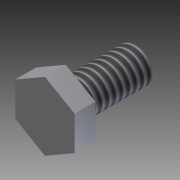
# Autodesk Inventor part: Bolt .5 1764
Saved by Autodesk Inventor 2011 (Build 150239000, 239)
## iProperties
Created: 2010-01-27
Part Number: Bolt .5 1764
Document SubType Name: Modeling
Designer: jgehrig
Density: 1 g/cm^3
Author: jgehrig
Autodesk Inventor part; units mm, degrees
ref_plane "YZ Plane" through (0, 0, 0) normal (1, 0, 0) x (0, 1, 0)
ref_plane "XZ Plane" through (0, 0, 0) normal (0, 1, 0) x (-1, 0, 0)
ref_plane "XY Plane" through (0, 0, 0) normal (0, 0, 1) x (1, 0, 0)
sketch "Sketch1" plane through (0, 0, 0) normal (0, 0, 1) x (1, 0, 0)
  circle A0 centre (0, 0) radius 3.175
  dimension "d0" = 6.35
  constraints: 1 centre point, 1 coincident
  measures "d0" diameter of A0
extrude "Extrusion1" add sketch "Sketch1" along normal blind 12.7
sketch "Sketch2" plane through (0, 0, 12.7) normal (0, 0, 1) x (1, 0, 0)
  circle A0 centre (0, 0) radius 3.175 projected
  line L0 (0, 6.2325) -> (5.3975, 3.1162)
  line L1 (5.3975, 3.1162) -> (5.3975, -3.1162)
  line L2 (5.3975, -3.1162) -> (0, -6.2325)
  line L3 (0, -6.2325) -> (-5.3975, -3.1162)
  line L4 (-5.3975, -3.1162) -> (-5.3975, 3.1162)
  line L5 (-5.3975, 3.1162) -> (0, 6.2325)
  dimension "d3" = 10.795
  constraints: 12 end point, 1 coincident, 13 other
  measures "d3" distance between parallel lines of L1 L4
extrude "Extrusion2" add sketch "Sketch2" along normal blind 3.81 contours A0 | L0 L1 L2 L3 L4 L5
thread "Thread1" size "1/4-20 UNC" class "2A" standard "ANSI Unified Screw Threads" full length
body "Solid1"
